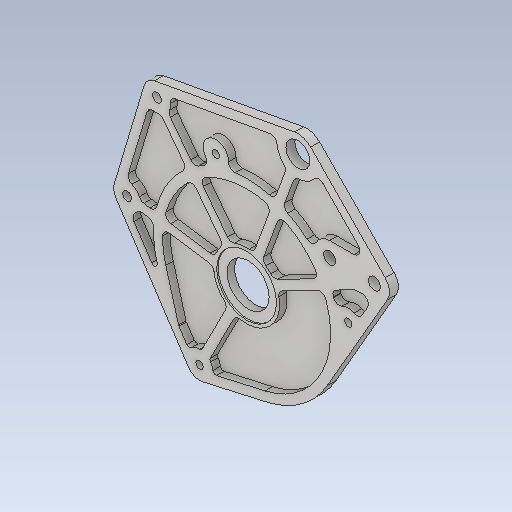
# Autodesk Inventor part: 前足内フレーム
Saved by Autodesk Inventor 2020 (Build 240168000, 168)
## iProperties
Created: 2019-09-17
Part Number: 前足内フレーム
Material: アルミニウム 2014-T4
Document SubType Name: Modeling
Designer: tanjihayato
Density: 2.8 g/cm^3
Appearance: サテン
Mass: 23.3541 g
Surface Area: 136.725 cm^2
Volume: 8.34073 cm^3
Author: tanjihayato
Autodesk Inventor part; units mm, degrees
note: some values were not read from the file. Chosen so that the rebuilt part matches the saved one: sketch regions of "押し出し9".
(part 1 of 2)
ref_plane "YZ Plane" through (0, 0, 0) normal (1, 0, 0) x (0, 1, 0)
ref_plane "XZ Plane" through (0, 0, 0) normal (0, 1, 0) x (-1, 0, 0)
ref_plane "XY Plane" through (0, 0, 0) normal (0, 0, 1) x (1, 0, 0)
sketch "スケッチ3" plane through (0, 0, 0) normal (0, 0, 1) x (1, 0, 0)
  circle A0 centre (110.4743, -16.4118) radius 30.1 construction
  circle A1 centre (150.4743, 0.5882) radius 1.5
  circle A2 centre (127.6431, 30.2622) radius 1.5
  circle A3 centre (80.4743, 23.124) radius 1.5
  circle A4 centre (70.4743, -10.4118) radius 1.5
  circle A5 centre (110.4743, -16.4118) radius 7.025
  arc A6 (79.801, 27.5733) -> (76.162, 24.4099) centre (80.4743, 23.124) ccw
  arc A7 (131.2097, 33.0062) -> (126.9698, 34.7115) centre (127.6431, 30.2622) ccw
  arc A8 (154.401, -1.6098) -> (154.0408, 3.3323) centre (150.4743, 0.5882) ccw
  arc A9 (66.162, -9.1259) -> (66.7172, -12.8885) centre (70.4743, -10.4118) ccw
  arc A10 (117.3199, -46.749) -> (137.6119, -31.6026) centre (110.4743, -16.4118) ccw
  line L0 (154.401, -1.6098) -> (137.6119, -31.6026)
  line L1 (66.162, -9.1259) -> (76.162, 24.4099)
  line L2 (79.801, 27.5733) -> (126.9698, 34.7115)
  line L3 (131.2097, 33.0062) -> (154.0408, 3.3323)
  line L4 (96.5433, 16.3458) -> (118.2214, -10.0492) construction
  line L5 (117.0311, -23.9953) -> (91.1935, -46.3348) construction
  circle A11 centre (100.1953, 16.6261) radius 3 construction
  circle A12 centre (144.4932, -10.0968) radius 3 construction
  circle A13 centre (100.1953, 16.6261) radius 4.5 construction
  circle A14 centre (144.4932, -10.0968) radius 4.5 construction
  arc A15 (90.988, -49.7066) -> (95.7356, -51.6195) centre (94.7451, -47.2298) ccw
  circle A16 centre (94.7451, -47.2298) radius 3 construction
  line L6 (95.7356, -51.6195) -> (117.3199, -46.749)
  line L7 (66.7172, -12.8885) -> (90.988, -49.7066)
  circle A17 centre (100.1953, 16.6261) radius 1.25
  circle A18 centre (144.4932, -10.0968) radius 1.25
  circle A19 centre (94.7451, -47.2298) radius 1.25
  circle A20 centre (110.4743, -16.4118) radius 30.1 construction
  circle A21 centre (150.4743, 0.5882) radius 1.5
  circle A22 centre (127.6431, 30.2622) radius 1.5
  circle A23 centre (80.4743, 23.124) radius 1.5
  circle A24 centre (70.4743, -10.4118) radius 1.5
  circle A25 centre (110.4743, -16.4118) radius 7.025
  arc A26 (79.801, 27.5733) -> (76.162, 24.4099) centre (80.4743, 23.124) ccw
  arc A27 (131.2097, 33.0062) -> (126.9698, 34.7115) centre (127.6431, 30.2622) ccw
  arc A28 (154.401, -1.6098) -> (154.0408, 3.3323) centre (150.4743, 0.5882) ccw
  arc A29 (66.162, -9.1259) -> (66.7172, -12.8885) centre (70.4743, -10.4118) ccw
  arc A30 (117.3199, -46.749) -> (137.6119, -31.6026) centre (110.4743, -16.4118) ccw
  line L8 (154.401, -1.6098) -> (137.6119, -31.6026)
  line L9 (66.162, -9.1259) -> (76.162, 24.4099)
  line L10 (79.801, 27.5733) -> (126.9698, 34.7115)
  line L11 (131.2097, 33.0062) -> (154.0408, 3.3323)
  line L12 (96.5433, 16.3458) -> (118.2214, -10.0492) construction
  line L13 (117.0311, -23.9953) -> (91.1935, -46.3348) construction
  circle A31 centre (100.1953, 16.6261) radius 3 construction
  circle A32 centre (144.4932, -10.0968) radius 3 construction
  circle A33 centre (100.1953, 16.6261) radius 4.5 construction
  circle A34 centre (144.4932, -10.0968) radius 4.5 construction
  arc A35 (90.988, -49.7066) -> (95.7356, -51.6195) centre (94.7451, -47.2298) ccw
  circle A36 centre (94.7451, -47.2298) radius 3 construction
  line L14 (95.7356, -51.6195) -> (117.3199, -46.749)
  line L15 (66.7172, -12.8885) -> (90.988, -49.7066)
  circle A37 centre (100.1953, 16.6261) radius 1.25
  circle A38 centre (144.4932, -10.0968) radius 1.25
  circle A39 centre (94.7451, -47.2298) radius 1.25
  circle A40 centre (153.2732, 5.5882) radius 1.5
  circle A41 centre (138.2732, 5.5882) radius 1.5
  arc A42 (157.1998, 3.3902) -> (156.3941, 8.8301) centre (153.2732, 5.5882) ccw
  line L16 (154.401, -1.6098) -> (157.1998, 3.3902)
  line L17 (130.7641, 33.504) -> (156.3941, 8.8301)
  circle A43 centre (138.2732, 5.5882) radius 3
  circle A44 centre (153.2732, 5.5882) radius 3
  point P0 (0, 0)
  point P1 (0, 0)
  point P2 (0, 0)
  dimension "d20" = 14.05
  dimension "d21" = 9
  dimension "d22" = 9
  dimension "d23" = 9
  dimension "d24" = 9
  dimension "d25" = 1
  dimension "d26" = 6
  dimension "d27" = 6
  dimension "d28" = 9
  dimension "d29" = 9
  dimension "d30" = 9
  dimension "d31" = 6
  dimension "d32" = 2.5
  dimension "d33" = 2.5
  dimension "d34" = 2.5
  dimension "d37" = 14.05
  dimension "d38" = 9
  dimension "d39" = 9
  dimension "d40" = 9
  dimension "d41" = 9
  dimension "d42" = 1
  dimension "d43" = 6
  dimension "d44" = 6
  dimension "d45" = 9
  dimension "d46" = 9
  dimension "d47" = 9
  dimension "d48" = 6
  dimension "d49" = 2.5
  dimension "d50" = 2.5
  dimension "d51" = 2.5
  dimension "d52" = 3
  dimension "d53" = 3
  dimension "d54" = 15
  dimension "d55" = 9
  dimension "d56" = 6
  dimension "d57" = 6
  dimension "d58" = 5
  constraints: 45 centre point, 39 tangent, 36 end point, 27 coincident, 27 point on circle, 1 collinear, 1 horizontal alignment
  measures "d20" diameter of A5
  measures "d21" diameter of A6
  measures "d22" diameter of A7
  measures "d23" diameter of A8
  measures "d24" diameter of A9
  measures "d25" radial gap between concentric circles of A10 A0
  measures "d26" diameter of A11
  measures "d27" diameter of A12
  measures "d28" diameter of A13
  measures "d29" diameter of A14
  measures "d30" diameter of A15
  measures "d31" diameter of A16
  measures "d32" diameter of A17
  measures "d33" diameter of A18
  measures "d34" diameter of A19
  measures "d37" diameter of A25
  measures "d38" diameter of A26
  measures "d39" diameter of A27
  measures "d40" diameter of A28
  measures "d41" diameter of A29
  measures "d42" radial gap between concentric circles of A30 A20
  measures "d43" diameter of A31
  measures "d44" diameter of A32
  measures "d45" diameter of A33
  measures "d46" diameter of A34
  measures "d47" diameter of A35
  measures "d48" diameter of A36
  measures "d49" diameter of A37
  measures "d50" diameter of A38
  measures "d51" diameter of A39
  measures "d52" diameter of A40
  measures "d53" diameter of A41
  measures "d54" distance of A41.centre A40.centre
  measures "d55" diameter of A42
  measures "d56" diameter of A43
  measures "d57" diameter of A44
  measures "d58" vertical distance of A21.centre A40.centre
extrude "押し出し3" add sketch "スケッチ3" along normal blind 3 contours A1 | L2 A7 L3 A44 A8 L0 A10 L6 A15 L7 A9 L1 A6 | L17 A42 L16 A8 A44 L3 A7 | A44 A8 L3 A40 | L3 A40 A8 A44 | A40 L3 | L3 A40 | A43
extrude "押し出し4" cut sketch "スケッチ3" along normal blind 10 contours A40 L3 | L3 A40
sketch "スケッチ4" plane through (0, 0, 3) normal (0, 0, 1) x (1, 0, 0)
  circle A0 centre (153.2732, 5.5882) radius 1.5 projected
  circle A1 centre (138.2732, 5.5882) radius 1.5 projected
  circle A2 centre (110.4743, -16.4118) radius 7.025 projected
  circle A3 centre (70.4743, -10.4118) radius 1.5 projected
  circle A4 centre (80.4743, 23.124) radius 1.5 projected
  circle A5 centre (127.6431, 30.2622) radius 1.5 projected
  circle A6 centre (94.7451, -47.2298) radius 1.25 projected
  circle A7 centre (144.4932, -10.0968) radius 1.25 projected
  circle A8 centre (100.1953, 16.6261) radius 1.25 projected
  arc A9 (79.801, 27.5733) -> (76.162, 24.4099) centre (80.4743, 23.124) ccw projected
  line L0 (76.162, 24.4099) -> (66.162, -9.1259) projected
  arc A10 (66.162, -9.1259) -> (66.7172, -12.8885) centre (70.4743, -10.4118) ccw projected
  line L1 (66.7172, -12.8885) -> (90.988, -49.7066) projected
  arc A11 (90.988, -49.7066) -> (95.7356, -51.6195) centre (94.7451, -47.2298) ccw projected
  line L2 (95.7356, -51.6195) -> (117.3199, -46.749) projected
  arc A12 (117.3199, -46.749) -> (137.6119, -31.6026) centre (110.4743, -16.4118) ccw projected
  line L3 (137.6119, -31.6026) -> (157.1998, 3.3902) projected
  arc A13 (157.1998, 3.3902) -> (156.3941, 8.8301) centre (153.2732, 5.5882) ccw projected
  line L4 (156.3941, 8.8301) -> (130.7641, 33.504) projected
  arc A14 (130.7641, 33.504) -> (126.9698, 34.7115) centre (127.6431, 30.2622) ccw projected
  line L5 (126.9698, 34.7115) -> (79.801, 27.5733) projected
  circle A15 centre (127.6431, 30.2622) radius 4.025
  arc A16 (131.983, 34.4054) -> (126.5593, 36.1635) centre (127.6431, 30.2622) ccw
  line L6 (79.6614, 27.5499) -> (126.5593, 36.1635)
  line L7 (131.983, 34.4054) -> (156.528, 8.6956)
  point P0 (0, 0)
  dimension "d61" = 8.05
  dimension "d62" = 12
  constraints: 4 end point, 4 point on circle, 4 tangent, 2 centre point, 2 coincident
  measures "d61" diameter of A15
  measures "d62" diameter of A16
extrude "押し出し5" add sketch "スケッチ4" against normal blind 3 contours A9 L6 A16 L7 A13 L4 A14 L5
extrude "押し出し6" cut sketch "スケッチ4" against normal blind 3 contours A15
sketch "スケッチ5" plane through (0, 0, 3) normal (0, 0, 1) x (1, 0, 0)
  circle A0 centre (127.6431, 30.2622) radius 4.025 projected
  circle A1 centre (153.2732, 5.5882) radius 1.5 projected
  circle A2 centre (138.2732, 5.5882) radius 1.5 projected
  circle A3 centre (110.4743, -16.4118) radius 7.025 projected
  circle A4 centre (70.4743, -10.4118) radius 1.5 projected
  circle A5 centre (80.4743, 23.124) radius 1.5 projected
  circle A6 centre (94.7451, -47.2298) radius 1.25 projected
  circle A7 centre (144.4932, -10.0968) radius 1.25 projected
  circle A8 centre (100.1953, 16.6261) radius 1.25 projected
  arc A9 (79.6614, 27.5499) -> (76.162, 24.4099) centre (80.4743, 23.124) ccw projected
  line L0 (76.162, 24.4099) -> (66.162, -9.1259) projected
  arc A10 (66.162, -9.1259) -> (66.7172, -12.8885) centre (70.4743, -10.4118) ccw projected
  line L1 (66.7172, -12.8885) -> (90.988, -49.7066) projected
  arc A11 (90.988, -49.7066) -> (95.7356, -51.6195) centre (94.7451, -47.2298) ccw projected
  line L2 (95.7356, -51.6195) -> (117.3199, -46.749) projected
  arc A12 (117.3199, -46.749) -> (137.6119, -31.6026) centre (110.4743, -16.4118) ccw projected
  line L3 (137.6119, -31.6026) -> (157.1998, 3.3902) projected
  arc A13 (157.1998, 3.3902) -> (156.528, 8.6956) centre (153.2732, 5.5882) ccw projected
  line L4 (156.528, 8.6956) -> (131.983, 34.4054) projected
  arc A14 (131.983, 34.4054) -> (126.5593, 36.1635) centre (127.6431, 30.2622) ccw projected
  line L5 (126.5593, 36.1635) -> (79.6614, 27.5499) projected
  circle A15 centre (153.2732, 5.5882) radius 2
  circle A16 centre (138.2732, 5.5882) radius 2
  arc A17 (157.6055, 3.092) -> (156.8408, 9.0914) centre (153.2732, 5.5882) ccw
  line L6 (131.9243, 34.466) -> (156.8408, 9.0914)
  line L7 (157.6055, 3.092) -> (137.4212, -31.9384)
  arc A18 (117.3199, -46.749) -> (137.6119, -31.6026) centre (110.4743, -16.4118) ccw projected
  arc A19 (131.983, 34.4054) -> (126.5593, 36.1635) centre (127.6431, 30.2622) ccw projected
  point P0 (0, 0)
  dimension "d67" = 4
  dimension "d68" = 4
  dimension "d69" = 3
  constraints: 4 end point, 4 point on circle, 4 tangent, 3 centre point, 2 coincident
  measures "d67" diameter of A15
  measures "d68" diameter of A16
  measures "d69" radial gap between concentric circles of A15 A17
extrude "押し出し7" add sketch "スケッチ5" against normal blind 3 contours L6 A17 L7 A12 L3 A13 L4
extrude "押し出し8" cut sketch "スケッチ5" against normal blind 3 contours A15 | A16
sketch "スケッチ6" plane through (0, 0, 3) normal (0, 0, 1) x (1, 0, 0)
  circle A0 centre (153.2732, 5.5882) radius 2 projected
  circle A1 centre (138.2732, 5.5882) radius 2 projected
  circle A2 centre (127.6431, 30.2622) radius 4.025 projected
  circle A3 centre (110.4743, -16.4118) radius 7.025 projected
  circle A4 centre (70.4743, -10.4118) radius 1.5 projected
  circle A5 centre (80.4743, 23.124) radius 1.5 projected
  circle A6 centre (94.7451, -47.2298) radius 1.25 projected
  circle A7 centre (144.4932, -10.0968) radius 1.25 projected
  circle A8 centre (100.1953, 16.6261) radius 1.25 projected
  arc A9 (79.6614, 27.5499) -> (76.162, 24.4099) centre (80.4743, 23.124) ccw projected
  line L0 (76.162, 24.4099) -> (66.162, -9.1259) projected
  arc A10 (66.162, -9.1259) -> (66.7172, -12.8885) centre (70.4743, -10.4118) ccw projected
  line L1 (66.7172, -12.8885) -> (90.988, -49.7066) projected
  arc A11 (90.988, -49.7066) -> (95.7356, -51.6195) centre (94.7451, -47.2298) ccw projected
  line L2 (95.7356, -51.6195) -> (117.3199, -46.749) projected
  arc A12 (117.3199, -46.749) -> (137.4212, -31.9384) centre (110.4743, -16.4118) ccw projected
  line L3 (137.4212, -31.9384) -> (157.6055, 3.092) projected
  arc A13 (157.6055, 3.092) -> (156.8408, 9.0914) centre (153.2732, 5.5882) ccw projected
  line L4 (156.8408, 9.0914) -> (131.9243, 34.466) projected
  arc A14 (131.9243, 34.466) -> (126.5593, 36.1635) centre (127.6431, 30.2622) ccw projected
  line L5 (126.5593, 36.1635) -> (79.6614, 27.5499) projected
  arc A15 (120.8535, 32.0653) -> (134.2343, 27.8317) centre (127.6431, 30.2622) ccw
  arc A16 (77.8245, 19.4869) -> (84.3762, 25.3657) centre (80.4743, 23.124) ccw
  arc A17 (71.557, -14.7796) -> (70.2492, -5.9174) centre (70.4743, -10.4118) ccw
  arc A18 (98.9543, -47.8178) -> (91.3042, -44.7354) centre (94.7451, -47.2298) ccw
  line L6 (153.2732, 5.5882) -> (138.2732, 5.5882) construction
  line L7 (151.1665, 10.5882) -> (138.2732, 10.5882)
  line L8 (138.2732, 0.5882) -> (152.7005, 0.5882)
  arc A19 (138.2732, 10.5882) -> (138.2732, 0.5882) centre (138.2732, 5.5882) ccw
  arc A20 (80.2034, 24.5993) -> (79.0369, 23.5526) centre (80.4743, 23.124) ccw
  line L9 (79.0369, 23.5526) -> (69.0369, -9.9832)
  arc A21 (69.0369, -9.9832) -> (69.222, -11.2374) centre (70.4743, -10.4118) ccw
  line L10 (69.222, -11.2374) -> (93.4928, -48.0554)
  arc A22 (93.4928, -48.0554) -> (95.0753, -48.6931) centre (94.7451, -47.2298) ccw
  line L11 (95.0753, -48.6931) -> (116.6595, -43.8226)
  arc A23 (116.6595, -43.8226) -> (134.8218, -30.4407) centre (110.4743, -16.4118) ccw
  line L12 (134.8218, -30.4407) -> (155.0061, 4.5897)
  arc A24 (155.0061, 4.5897) -> (154.7002, 6.9895) centre (153.2732, 5.5882) ccw
  line L13 (154.7002, 6.9895) -> (129.7837, 32.3641)
  arc A25 (129.7837, 32.3641) -> (127.1012, 33.2128) centre (127.6431, 30.2622) ccw
  line L14 (127.1012, 33.2128) -> (80.2034, 24.5993)
  circle A26 centre (100.1953, 16.6261) radius 4.25
  circle A27 centre (144.4932, -10.0968) radius 4.25
  circle A28 centre (110.4743, -16.4118) radius 11.025
  circle A29 centre (110.4743, -16.4118) radius 31.1
  circle A30 centre (110.4743, -16.4118) radius 28.1
  line L15 (127.6431, 30.2622) -> (110.4743, -16.4118) construction
  arc A31 (129.0509, 29.7443) -> (126.2354, 30.78) centre (127.6431, 30.2622) ccw
  arc A32 (109.0666, -15.894) -> (111.8821, -16.9296) centre (110.4743, -16.4118) ccw
  line L16 (80.4743, 23.124) -> (110.4743, -16.4118) construction
  arc A33 (81.6693, 24.0307) -> (79.2794, 22.2173) centre (80.4743, 23.124) ccw
  arc A34 (109.2794, -17.3185) -> (111.6693, -15.5051) centre (110.4743, -16.4118) ccw
  line L17 (94.7451, -47.2298) -> (110.4743, -16.4118) construction
  arc A35 (93.4091, -46.5479) -> (96.0812, -47.9118) centre (94.7451, -47.2298) ccw
  arc A36 (111.8104, -17.0937) -> (109.1383, -15.7299) centre (110.4743, -16.4118) ccw
  line L18 (153.2732, 5.5882) -> (110.4743, -16.4118) construction
  arc A37 (153.9589, 4.2541) -> (152.5874, 6.9223) centre (153.2732, 5.5882) ccw
  arc A38 (109.7886, -15.0777) -> (111.1601, -17.7459) centre (110.4743, -16.4118) ccw
  line L19 (70.4743, -10.4118) -> (110.4743, -16.4118) construction
  arc A39 (70.6968, -8.9284) -> (70.2518, -11.8952) centre (70.4743, -10.4118) ccw
  arc A40 (110.2518, -17.8952) -> (110.6968, -14.9284) centre (110.4743, -16.4118) ccw
  line L20 (111.1601, -17.7459) -> (111.5904, -17.5247)
  line L21 (117.2639, -14.6083) -> (153.9589, 4.2541)
  line L22 (152.5874, 6.9223) -> (115.8924, -11.9402)
  line L23 (113.2103, -13.3188) -> (109.7886, -15.0777)
  line L24 (111.8821, -16.9296) -> (113.2103, -13.3188)
  line L25 (114.2514, -10.4886) -> (129.0509, 29.7443)
  line L26 (126.2354, 30.78) -> (111.4359, -9.4529)
  line L27 (110.0127, -13.3219) -> (109.0666, -15.894)
  line L28 (111.6693, -15.5051) -> (110.0127, -13.3219)
  line L29 (107.5207, -10.0379) -> (81.6693, 24.0307)
  line L30 (79.2794, 22.2173) -> (105.1309, -11.8513)
  line L31 (107.0508, -14.3815) -> (109.2794, -17.3185)
  line L32 (110.6968, -14.9284) -> (107.0508, -14.3815)
  line L33 (103.9098, -13.9103) -> (70.6968, -8.9284)
  line L34 (70.2518, -11.8952) -> (103.4648, -16.8771)
  line L35 (108.1909, -17.5861) -> (110.2518, -17.8952)
  line L36 (109.1383, -15.7299) -> (108.1909, -17.5861)
  line L37 (106.0184, -21.8427) -> (93.4091, -46.5479)
  line L38 (96.0812, -47.9118) -> (108.6904, -23.2065)
  line L39 (111.5904, -17.5247) -> (111.8104, -17.0937)
  circle A41 centre (110.4743, -16.4118) radius 10
  point P0 (0, 0)
  point P1 (145.7732, 5.5882)
  point P2 (119.0587, 6.9252)
  point P3 (95.4743, 3.3561)
  point P4 (102.6097, -31.8208)
  point P5 (131.8738, -5.4118)
  point P6 (90.4743, -13.4118)
  dimension "d74" = 10
  dimension "d75" = 3
  dimension "d76" = 3
  dimension "d77" = 3
  dimension "d78" = 3
  dimension "d79" = 3
  dimension "d80" = 3
  dimension "d81" = 3
  dimension "d82" = 4
  dimension "d83" = 3
  dimension "d84" = 3
  dimension "d85" = 3
  dimension "d86" = 3
  dimension "d87" = 3
  dimension "d100" = 20
  constraints: 80 end point, 42 point on circle, 42 tangent, 27 centre point, 21 parallel, 10 point on line, 7 coincident, 6 midpoint, 5 concentric, 2 horizontal, 22 other
  measures "d74" diameter of A19
  measures "d75" distance between parallel lines of L5 L14
  measures "d76" radial gap between concentric circles of A8 A26
  measures "d77" radial gap between concentric circles of A7 A27
  measures "d78" radial gap between concentric circles of A16 A5
  measures "d79" radial gap between concentric circles of A17 A4
  measures "d80" radial gap between concentric circles of A18 A6
  measures "d81" radial gap between concentric circles of A15 A2
  measures "d83" diameter of A32
  measures "d84" diameter of A34
  measures "d85" diameter of A36
  measures "d86" diameter of A38
  measures "d87" diameter of A40
  measures "d100" diameter of A41
extrude "押し出し9" cut sketch "スケッチ6" against normal blind 10 contours L7 A19 A29 L25 A15 L13 | L12 A27 A29 L21 L8 | L22 A29 A19 L8 | L8 L21 A29 L22 | L12 A27 A29 | L22 A30 L25 A29 A19 | A29 L21 A30 L22 | L25 A29 L26 A15 | A29 A27 L12 A30 L21 | L12 A29 A27 | A29 A27 | L22 A28 L25 A30 | A30 L21 A28 L22 | L25 A30 L26 A29 | L26 A29 A26 L29 A16 L14 A15 | A30 A23 L38 A28 L21 | L25 A28 L26 A30 | L26 A30 L29 A29 A26 | L26 A28 L29 A30 | L11 A29 A18 L38 A30 | L29 A28 L30 A30 | A30 L30 A29 L29 | L29 A29 L30 A16 | L38 A30 L37 A28 | L11 A18 A29 | L38 A18 L37 A30 | L30 A28 L33 A30 | A30 L33 A29 L30 | L30 A29 L33 A17 L9 A16 | L37 A30 L34 A28 | L37 A18 A29 L34 A30 | L33 A28 L34 A30 | A30 L34 A29 L33 | A29 L34 A17 L33 | A29 A18 L10 A17 L34
extrude "押し出し10" add sketch "スケッチ6" against normal blind 3 contours L22 A37 L21 A0 | A0 L21 L8 L22 | L8 L21 A29 L22 | A27 L12 | L12 A27 A29 | L22 A30 L25 A29 A19 | A29 L21 A30 L22 | A29 A19 | L25 A29 L26 A15 | A15 L26 A2 L25 | A29 A27 L12 A30 L21 | A29 A27 | A30 L21 A28 L22 | L25 A30 L26 A29 | A2 L26 A31 L25 | A29 A12 L11 A23 L12 | L25 A28 L26 A30 | A28 L21 A41 L22 | L26 A30 L29 A29 A26 | L25 A41 L26 A28 | A41 L21 A3 L22 | A26 A29 | L11 A29 A18 L38 A30 | L29 A28 L30 A30 | A30 L30 A29 L29 | L25 A3 L26 A41 | L29 A29 L30 A16 | A16 L30 A5 L29 | L38 A30 L37 A28 | A28 L37 A41 L38 | L38 A18 L37 A30 | A30 L33 A29 L30 | L29 A41 L30 A28 | A41 L37 A3 L38 | A29 L38 A18 | L37 A18 A29 L34 A30 | L38 A29 L37 A18 | L33 A28 L34 A30 | A30 L34 A29 L33 | L29 A3 L30 A41 | A28 L33 A41 L34 | A22 A35 L37 A29 L38 | L37 A29 A18 | A29 L34 A17 L33 | A41 L33 A3 L34 | A17 L34 A4 L33 picked at (152.6478, 5.3573) picked at (145.8885, -10.8818) picked at (101.4617, 13.0958)
extrude "押し出し11" cut sketch "スケッチ6" against normal blind 3 contours A0 L21 A37 L22 | L22 A37 L21 A0 | L13 A25 L14 A2 | A2 L25 A31 L26 L14 A25 L13 | A2 L26 A31 L25
sketch "スケッチ7" plane through (0, 0, 3) normal (0, 0, 1) x (1, 0, 0)
  circle A0 centre (153.2732, 5.5882) radius 2 projected
  circle A1 centre (127.6431, 30.2622) radius 4.025 projected
  line L0 (144.1052, -14.3291) -> (141.4751, -18.8937) projected
  arc A2 (141.4751, -18.8937) -> (141.3863, -12.9968) centre (110.4743, -16.4118) ccw projected
  arc A3 (141.3863, -12.9968) -> (144.1052, -14.3291) centre (144.4932, -10.0968) ccw projected
  arc A4 (136.2251, 1.0269) -> (138.2732, 0.5882) centre (138.2732, 5.5882) ccw projected
  line L1 (138.2732, 0.5882) -> (140.2651, 0.5882) projected
  line L2 (140.2651, 0.5882) -> (137.4161, -0.8763) projected
  arc A5 (137.4161, -0.8763) -> (136.2251, 1.0269) centre (110.4743, -16.4118) ccw projected
  arc A6 (94.3399, -42.9992) -> (91.3042, -44.7354) centre (94.7451, -47.2298) ccw projected
  line L3 (91.3042, -44.7354) -> (71.557, -14.7796) projected
  arc A7 (71.557, -14.7796) -> (74.4475, -12.5246) centre (70.4743, -10.4118) ccw projected
  line L4 (74.4475, -12.5246) -> (79.5317, -13.2872) projected
  arc A8 (79.5317, -13.2872) -> (94.3399, -42.9992) centre (110.4743, -16.4118) ccw projected
  arc A9 (147.9602, -7.6387) -> (140.5525, -8.5052) centre (144.4932, -10.0968) ccw projected
  arc A10 (140.5525, -8.5052) -> (138.7876, -3.5444) centre (110.4743, -16.4118) ccw projected
  line L5 (138.7876, -3.5444) -> (146.8272, 0.5882) projected
  line L6 (146.8272, 0.5882) -> (152.7005, 0.5882) projected
  line L7 (152.7005, 0.5882) -> (147.9602, -7.6387) projected
  arc A11 (99.0543, -42.0865) -> (136.116, -4.9177) centre (110.4743, -16.4118) ccw projected
  line L8 (99.0543, -42.0865) -> (106.845, -26.8223) projected
  arc A12 (106.845, -26.8223) -> (120.8743, -12.7524) centre (110.4743, -16.4118) ccw projected
  line L9 (120.8743, -12.7524) -> (136.116, -4.9177) projected
  arc A13 (98.4089, -45.076) -> (103.6597, -46.756) centre (110.4743, -16.4118) ccw projected
  line L10 (103.6597, -46.756) -> (98.9543, -47.8178) projected
  arc A14 (98.9543, -47.8178) -> (98.4089, -45.076) centre (94.7451, -47.2298) ccw projected
  arc A15 (133.3633, 4.643) -> (122.6063, 12.2243) centre (110.4743, -16.4118) ccw projected
  line L11 (122.6063, 12.2243) -> (126.6816, 23.3033) projected
  arc A16 (126.6816, 23.3033) -> (134.2343, 27.8317) centre (127.6431, 30.2622) ccw projected
  line L12 (134.2343, 27.8317) -> (151.1665, 10.5882) projected
  line L13 (151.1665, 10.5882) -> (138.2732, 10.5882) projected
  arc A17 (138.2732, 10.5882) -> (133.3633, 4.643) centre (138.2732, 5.5882) ccw projected
  arc A18 (74.8925, -9.5578) -> (70.2492, -5.9174) centre (70.4743, -10.4118) ccw projected
  line L14 (70.2492, -5.9174) -> (77.8245, 19.4869) projected
  arc A19 (77.8245, 19.4869) -> (81.844, 18.8375) centre (80.4743, 23.124) ccw projected
  line L15 (81.844, 18.8375) -> (90.5019, 7.4275) projected
  arc A20 (90.5019, 7.4275) -> (79.9767, -10.3204) centre (110.4743, -16.4118) ccw projected
  line L16 (79.9767, -10.3204) -> (74.8925, -9.5578) projected
  line L17 (104.1729, -25.4585) -> (96.3822, -40.7227) projected
  arc A21 (82.5023, -13.7328) -> (96.3822, -40.7227) centre (110.4743, -16.4118) ccw projected
  line L18 (82.5023, -13.7328) -> (99.4502, -16.275) projected
  arc A22 (99.4502, -16.275) -> (104.1729, -25.4585) centre (110.4743, -16.4118) ccw projected
  circle A23 centre (110.4743, -16.4118) radius 7.025 projected
  circle A24 centre (144.4932, -10.0968) radius 1.25 projected
  circle A25 centre (100.1953, 16.6261) radius 1.25 projected
  arc A26 (102.677, -8.6175) -> (99.8952, -13.3081) centre (110.4743, -16.4118) ccw projected
  line L19 (99.8952, -13.3081) -> (82.9474, -10.766) projected
  arc A27 (92.3177, 5.0346) -> (82.9474, -10.766) centre (110.4743, -16.4118) ccw projected
  line L20 (92.3177, 5.0346) -> (102.677, -8.6175) projected
  line L21 (115.6529, -6.6787) -> (121.5692, 9.4051) projected
  arc A28 (134.7445, -2.2496) -> (121.5692, 9.4051) centre (110.4743, -16.4118) ccw projected
  line L22 (134.7445, -2.2496) -> (119.5028, -10.0843) projected
  arc A29 (119.5028, -10.0843) -> (115.6529, -6.6787) centre (110.4743, -16.4118) ccw projected
  arc A30 (112.8373, -5.643) -> (105.0668, -6.804) centre (110.4743, -16.4118) ccw projected
  line L23 (105.0668, -6.804) -> (94.7076, 6.848) projected
  arc A31 (118.7537, 10.4408) -> (94.7076, 6.848) centre (110.4743, -16.4118) ccw projected
  line L24 (118.7537, 10.4408) -> (112.8373, -5.643) projected
  circle A32 centre (94.7451, -47.2298) radius 1.25 projected
  line L25 (123.8661, 24.339) -> (119.7907, 13.26) projected
  arc A33 (119.7907, 13.26) -> (103.4411, 13.8825) centre (110.4743, -16.4118) ccw projected
  arc A34 (103.4411, 13.8825) -> (99.079, 12.5253) centre (100.1953, 16.6261) ccw projected
  arc A35 (99.079, 12.5253) -> (92.8918, 9.241) centre (110.4743, -16.4118) ccw projected
  line L26 (92.8918, 9.241) -> (84.2339, 20.6509) projected
  arc A36 (84.2339, 20.6509) -> (84.3762, 25.3657) centre (80.4743, 23.124) ccw projected
  line L27 (84.3762, 25.3657) -> (120.8535, 32.0653) projected
  arc A37 (120.8535, 32.0653) -> (123.8661, 24.339) centre (127.6431, 30.2622) ccw projected
  arc A38 (117.3199, -46.749) -> (137.4212, -31.9384) centre (110.4743, -16.4118) ccw projected
  line L28 (137.4212, -31.9384) -> (157.6055, 3.092) projected
  arc A39 (157.6055, 3.092) -> (156.8408, 9.0914) centre (153.2732, 5.5882) ccw projected
  line L29 (156.8408, 9.0914) -> (131.9243, 34.466) projected
  arc A40 (131.9243, 34.466) -> (126.5593, 36.1635) centre (127.6431, 30.2622) ccw projected
  line L30 (126.5593, 36.1635) -> (79.6614, 27.5499) projected
  arc A41 (79.6614, 27.5499) -> (76.162, 24.4099) centre (80.4743, 23.124) ccw projected
  line L31 (76.162, 24.4099) -> (66.162, -9.1259) projected
  arc A42 (66.162, -9.1259) -> (66.7172, -12.8885) centre (70.4743, -10.4118) ccw projected
  line L32 (66.7172, -12.8885) -> (90.988, -49.7066) projected
  arc A43 (90.988, -49.7066) -> (95.7356, -51.6195) centre (94.7451, -47.2298) ccw projected
  line L33 (95.7356, -51.6195) -> (117.3199, -46.749) projected
  circle A44 centre (80.4743, 23.124) radius 1.5 projected
  circle A45 centre (138.2732, 5.5882) radius 2 projected
  circle A46 centre (70.4743, -10.4118) radius 1.5 projected
  arc A47 (78.7483, -25.6886) -> (80.5456, -24.8663) centre (79.5832, -25.1382) ccw
  line L34 (91.3042, -44.7354) -> (71.557, -14.7796) projected
  point P0 (0, 0)
  dimension "d94" = 2
  constraints: 3 point on circle, 2 tangent, 1 centre point, 1 point on line
  measures "d94" diameter of A47
extrude "押し出し12" add sketch "スケッチ7" against normal blind 3 contours L0 A2 A3 | A4 L1 L2 A5 | A6 L3 A47 A8 | A13 L10 A14
fillet "フィレット1" radius 2 47 edges at (152.7005, 0.5882, 1.5) (147.9602, -7.6387, 1.5) (146.8272, 0.5882, 1.5) (133.3633, 4.643, 1.5) (151.1665, 10.5882, 1.5) (134.2343, 27.8317, 1.5) (126.6816, 23.3033, 1.5) (120.8535, 32.0653, 1.5) (123.8661, 24.339, 1.5) (84.3762, 25.3657, 1.5) (84.2339, 20.6509, 1.5) (77.8245, 19.4869, 1.5) (81.844, 18.8375, 1.5) (70.2492, -5.9174, 1.5) (74.8925, -9.5578, 1.5) (71.557, -14.7796, 1.5) (74.4475, -12.5246, 1.5) (140.5525, -8.5052, 1.5) (138.7876, -3.5444, 1.5) (122.6063, 12.2243, 1.5) (119.7907, 13.26, 1.5) (92.8918, 9.241, 1.5) (90.5019, 7.4275, 1.5) (79.9767, -10.3204, 1.5) (79.5317, -13.2872, 1.5) (136.116, -4.9177, 1.5) (120.8743, -12.7524, 1.5) (119.5028, -10.0843, 1.5) (134.7445, -2.2496, 1.5) (121.5692, 9.4051, 1.5) (115.6529, -6.6787, 1.5) (112.8373, -5.643, 1.5) (118.7537, 10.4408, 1.5) (94.7076, 6.848, 1.5) (105.0668, -6.804, 1.5) (102.677, -8.6175, 1.5) (92.3177, 5.0346, 1.5) (82.9474, -10.766, 1.5) (99.8952, -13.3081, 1.5) (99.4502, -16.275, 1.5) (82.5023, -13.7328, 1.5) (96.3822, -40.7227, 1.5) (104.1729, -25.4585, 1.5) (106.845, -26.8223, 1.5) (99.0543, -42.0865, 1.5) (99.079, 12.5253, 1.5) (103.4411, 13.8825, 1.5)
sketch "スケッチ8" plane through (0, 0, 0) normal (0, 0, -1) x (-1, 0, 0)
  line L0 (-149.151, -5.572) -> (-150.9727, -2.4103) projected
  arc A0 (-149.2398, 0.5882) -> (-150.9727, -2.4103) centre (-149.2398, -1.4118) ccw projected
  line L1 (-149.2398, 0.5882) -> (-147.3112, 0.5882) projected
  arc A1 (-146.3968, 0.367) -> (-147.3112, 0.5882) centre (-147.3112, -1.4118) ccw projected
  line L2 (-146.3968, 0.367) -> (-140.4335, -2.6984) projected
  arc A2 (-139.4824, -5.1983) -> (-140.4335, -2.6984) centre (-141.3478, -4.4771) ccw projected
  arc A3 (-139.4824, -5.1983) -> (-139.547, -5.3668) centre (-110.4743, -16.4118) ccw projected
  arc A4 (-142.4011, -6.3974) -> (-139.547, -5.3668) centre (-141.4166, -4.6565) ccw projected
  arc A5 (-142.4011, -6.3974) -> (-146.4821, -6.341) centre (-144.4932, -10.0968) ccw projected
  arc A6 (-149.151, -5.572) -> (-146.4821, -6.341) centre (-147.4181, -4.5735) ccw projected
  arc A7 (-133.802, 7.8261) -> (-138.2732, 10.5882) centre (-138.2732, 5.5882) ccw projected
  line L3 (-138.2732, 10.5882) -> (-146.3996, 10.5882) projected
  arc A8 (-147.8266, 13.9895) -> (-146.3996, 10.5882) centre (-146.3996, 12.5882) ccw projected
  line L4 (-147.8266, 13.9895) -> (-136.068, 25.9642) projected
  arc A9 (-133.0902, 25.8259) -> (-136.068, 25.9642) centre (-134.641, 24.563) ccw projected
  arc A10 (-133.0902, 25.8259) -> (-127.9646, 23.2445) centre (-127.6431, 30.2622) ccw projected
  arc A11 (-126.1791, 21.9371) -> (-127.9646, 23.2445) centre (-128.0561, 21.2466) ccw projected
  line L5 (-126.1791, 21.9371) -> (-123.2452, 13.9611) projected
  arc A12 (-124.2371, 11.4772) -> (-123.2452, 13.9611) centre (-125.1222, 13.2707) ccw projected
  arc A13 (-124.2371, 11.4772) -> (-130.712, 7.2027) centre (-110.4743, -16.4118) ccw projected
  arc A14 (-133.802, 7.8261) -> (-130.712, 7.2027) centre (-132.0135, 8.7213) ccw projected
  arc A15 (-136.9629, -7.0327) -> (-101.1717, -42.9273) centre (-110.4743, -16.4118) ccw projected
  arc A16 (-134.1632, -5.9215) -> (-136.9629, -7.0327) centre (-135.0776, -7.7003) ccw projected
  line L6 (-134.1632, -5.9215) -> (-122.3182, -12.0102) projected
  arc A17 (-121.2735, -14.1917) -> (-122.3182, -12.0102) centre (-123.2325, -13.789) ccw projected
  arc A18 (-121.2735, -14.1917) -> (-108.2854, -27.2173) centre (-110.4743, -16.4118) ccw projected
  arc A19 (-106.107, -28.2683) -> (-108.2854, -27.2173) centre (-107.8884, -29.1775) ccw projected
  line L7 (-106.107, -28.2683) -> (-100.0524, -40.1309) projected
  arc A20 (-101.1717, -42.9273) -> (-100.0524, -40.1309) centre (-101.8338, -41.0401) ccw projected
  arc A21 (-122.8508, 25.1256) -> (-120.6357, 29.7665) centre (-127.6431, 30.2622) ccw projected
  arc A22 (-118.2794, 31.5925) -> (-120.6357, 29.7665) centre (-118.6406, 29.6254) ccw projected
  line L8 (-118.2794, 31.5925) -> (-86.5775, 25.77) projected
  arc A23 (-84.9497, 23.594) -> (-86.5775, 25.77) centre (-86.9388, 23.8029) ccw projected
  arc A24 (-84.9497, 23.594) -> (-84.6967, 21.568) centre (-80.4743, 23.124) ccw projected
  arc A25 (-84.9801, 19.6674) -> (-84.6967, 21.568) centre (-86.5734, 20.8764) ccw projected
  line L9 (-84.9801, 19.6674) -> (-91.7731, 10.7152) projected
  arc A26 (-94.4001, 10.212) -> (-91.7731, 10.7152) centre (-93.3664, 11.9242) ccw projected
  arc A27 (-94.4001, 10.212) -> (-96.0809, 11.157) centre (-110.4743, -16.4118) ccw projected
  arc A28 (-96.7681, 14.1127) -> (-96.0809, 11.157) centre (-95.1553, 12.9299) ccw projected
  arc A29 (-96.7681, 14.1127) -> (-104.4434, 16.5007) centre (-100.1953, 16.6261) ccw projected
  arc A30 (-106.6862, 14.4566) -> (-104.4434, 16.5007) centre (-106.4426, 16.4417) ccw projected
  arc A31 (-106.6862, 14.4566) -> (-118.0645, 13.7478) centre (-110.4743, -16.4118) ccw projected
  arc A32 (-120.4296, 14.9968) -> (-118.0645, 13.7478) centre (-118.5526, 15.6873) ccw projected
  line L10 (-120.4296, 14.9968) -> (-123.3635, 22.9728) projected
  arc A33 (-122.8508, 25.1256) -> (-123.3635, 22.9728) centre (-121.4865, 23.6632) ccw projected
  arc A34 (-80.5456, -24.8663) -> (-79.403, -15.0764) centre (-110.4743, -16.4118) ccw projected
  arc A35 (-77.7015, -13.0127) -> (-79.403, -15.0764) centre (-77.4049, -14.9905) ccw projected
  line L11 (-77.7015, -13.0127) -> (-75.6684, -12.7077) projected
  arc A36 (-73.8649, -13.3706) -> (-75.6684, -12.7077) centre (-75.3718, -14.6856) ccw projected
  arc A37 (-73.8649, -13.3706) -> (-73.2327, -13.9673) centre (-70.4743, -10.4118) ccw projected
  arc A38 (-72.7888, -16.6482) -> (-73.2327, -13.9673) centre (-74.4587, -15.5475) ccw projected
  line L12 (-72.7888, -16.6482) -> (-78.7483, -25.6886) projected
  arc A39 (-80.5456, -24.8663) -> (-78.7483, -25.6886) centre (-79.5832, -25.1382) ccw projected
  circle A40 centre (-110.4743, -16.4118) radius 7.025 projected
  line L13 (-101.6956, -7.3242) -> (-93.645, 3.2855) projected
  arc A41 (-90.64, 3.4932) -> (-93.645, 3.2855) centre (-92.0517, 2.0765) ccw projected
  arc A42 (-83.4952, -8.5546) -> (-90.64, 3.4932) centre (-110.4743, -16.4118) ccw projected
  arc A43 (-85.1187, -11.0917) -> (-83.4952, -8.5546) centre (-85.4154, -9.1138) ccw projected
  line L14 (-85.1187, -11.0917) -> (-98.2897, -13.0673) projected
  arc A44 (-100.4118, -11.9067) -> (-98.2897, -13.0673) centre (-98.5864, -11.0895) ccw projected
  arc A45 (-100.4118, -11.9067) -> (-101.695, -9.7429) centre (-110.4743, -16.4118) ccw projected
  arc A46 (-101.6956, -7.3242) -> (-101.695, -9.7429) centre (-100.1024, -8.5331) ccw projected
  circle A47 centre (-144.4932, -10.0968) radius 1.25 projected
  circle A48 centre (-100.1953, 16.6261) radius 1.25 projected
  arc A49 (-103.0079, -24.5237) -> (-99.5329, -17.7663) centre (-110.4743, -16.4118) ccw projected
  arc A50 (-97.8447, -16.0341) -> (-99.5329, -17.7663) centre (-97.548, -18.012) ccw projected
  line L15 (-97.8447, -16.0341) -> (-84.6737, -14.0585) projected
  arc A51 (-82.3772, -16.0076) -> (-84.6737, -14.0585) centre (-84.377, -16.0364) ccw projected
  arc A52 (-94.4591, -39.5012) -> (-82.3772, -16.0076) centre (-110.4743, -16.4118) ccw projected
  arc A53 (-97.3804, -38.7671) -> (-94.4591, -39.5012) centre (-95.599, -37.8579) ccw projected
  line L16 (-97.3804, -38.7671) -> (-103.4349, -26.9045) projected
  arc A54 (-103.0079, -24.5237) -> (-103.4349, -26.9045) centre (-101.6535, -25.9953) ccw projected
  line L17 (-113.3978, -4.1194) -> (-117.9957, 8.3801) projected
  arc A55 (-116.5511, 11.0233) -> (-117.9957, 8.3801) centre (-116.1186, 9.0706) ccw projected
  arc A56 (-96.6437, 8.0488) -> (-116.5511, 11.0233) centre (-110.4743, -16.4118) ccw projected
  arc A57 (-96.0348, 5.0989) -> (-96.6437, 8.0488) centre (-97.6281, 6.3079) ccw projected
  line L18 (-96.0348, 5.0989) -> (-104.0855, -5.5107) projected
  arc A58 (-106.4151, -6.1613) -> (-104.0855, -5.5107) centre (-105.6787, -4.3018) ccw projected
  arc A59 (-106.4151, -6.1613) -> (-111.3601, -5.4224) centre (-110.4743, -16.4118) ccw projected
  arc A60 (-113.3978, -4.1194) -> (-111.3601, -5.4224) centre (-111.5208, -3.4289) ccw projected
  arc A61 (-116.9209, -7.468) -> (-118.5647, -8.922) centre (-110.4743, -16.4118) ccw projected
  arc A62 (-120.9467, -9.3421) -> (-118.5647, -8.922) centre (-120.0323, -7.5633) ccw projected
  line L19 (-120.9467, -9.3421) -> (-132.7917, -3.2534) projected
  arc A63 (-133.5175, -0.33) -> (-132.7917, -3.2534) centre (-131.8774, -1.4746) ccw projected
  arc A64 (-123.6242, 8.4215) -> (-133.5175, -0.33) centre (-110.4743, -16.4118) ccw projected
  arc A65 (-120.8112, 7.3444) -> (-123.6242, 8.4215) centre (-122.6883, 6.654) ccw projected
  line L20 (-120.8112, 7.3444) -> (-116.2133, -5.1551) projected
  arc A66 (-116.9209, -7.468) -> (-116.2133, -5.1551) centre (-118.0904, -5.8455) ccw projected
  circle A67 centre (-94.7451, -47.2298) radius 1.25 projected
  circle A68 centre (-153.2732, 5.5882) radius 2 projected
  line L21 (-76.1135, -9.7409) -> (-78.1466, -10.0459) projected
  arc A69 (-80.3787, -8.5721) -> (-78.1466, -10.0459) centre (-78.4432, -8.068) ccw projected
  arc A70 (-80.3787, -8.5721) -> (-89.1607, 6.2363) centre (-110.4743, -16.4118) ccw projected
  arc A71 (-89.3833, 8.9018) -> (-89.1607, 6.2363) centre (-87.79, 7.6928) ccw projected
  line L22 (-89.3833, 8.9018) -> (-82.5903, 17.854) projected
  arc A72 (-80.8362, 18.6385) -> (-82.5903, 17.854) centre (-80.997, 16.645) ccw projected
  arc A73 (-80.8362, 18.6385) -> (-79.524, 18.7255) centre (-80.4743, 23.124) ccw projected
  arc A74 (-77.185, 17.3421) -> (-79.524, 18.7255) centre (-79.1016, 16.7706) ccw projected
  line L23 (-77.185, 17.3421) -> (-70.8888, -3.7727) projected
  arc A75 (-72.0881, -6.2111) -> (-70.8888, -3.7727) centre (-72.8054, -4.3442) ccw projected
  arc A76 (-72.0881, -6.2111) -> (-74.5837, -8.578) centre (-70.4743, -10.4118) ccw projected
  arc A77 (-76.1135, -9.7409) -> (-74.5837, -8.578) centre (-76.4101, -7.763) ccw projected
  circle A78 centre (-127.6431, 30.2622) radius 4.025 projected
  circle A79 centre (-70.4743, -10.4118) radius 1.5 projected
  arc A80 (-137.4212, -31.9384) -> (-117.3199, -46.749) centre (-110.4743, -16.4118) ccw projected
  line L24 (-95.7356, -51.6195) -> (-117.3199, -46.749) projected
  arc A81 (-95.7356, -51.6195) -> (-90.988, -49.7066) centre (-94.7451, -47.2298) ccw projected
  line L25 (-66.7172, -12.8885) -> (-90.988, -49.7066) projected
  arc A82 (-66.7172, -12.8885) -> (-66.162, -9.1259) centre (-70.4743, -10.4118) ccw projected
  line L26 (-76.162, 24.4099) -> (-66.162, -9.1259) projected
  arc A83 (-76.162, 24.4099) -> (-79.6614, 27.5499) centre (-80.4743, 23.124) ccw projected
  line L27 (-79.6614, 27.5499) -> (-126.5593, 36.1635) projected
  arc A84 (-126.5593, 36.1635) -> (-131.9243, 34.466) centre (-127.6431, 30.2622) ccw projected
  line L28 (-131.9243, 34.466) -> (-156.8408, 9.0914) projected
  arc A85 (-156.8408, 9.0914) -> (-157.6055, 3.092) centre (-153.2732, 5.5882) ccw projected
  line L29 (-157.6055, 3.092) -> (-137.4212, -31.9384) projected
  circle A86 centre (-80.4743, 23.124) radius 1.5 projected
  circle A87 centre (-138.2732, 5.5882) radius 2 projected
  point P0 (0, 0)
extrude "押し出し13" add sketch "スケッチ8" against normal blind 0.5 contours L0 A0 L1 A1 L2 A2 A3 A4 A5 A6 | A7 L3 A8 L4 A9 A10 A11 L5 A12 A13 A14 | A16 L6 A17 A18 A19 L7 A20 A15 | A21 A22 L8 A23 A24 A25 L9 A26 A27 A28 A29 A30 A31 A32 L10 A33 | A34 A35 L11 A36 A37 A38 L12 A39 | L13 A41 A42 A43 L14 A44 A45 A46 | A49 A50 L15 A51 A52 A53 L16 A54 | L17 A55 A56 A57 L18 A58 A59 A60 | A61 A62 L19 A63 A64 A65 L20 A66 | L21 A69 A70 A71 L22 A72 A73 A74 L23 A75 A76 A77
extrude "押し出し14" cut sketch "スケッチ6" against normal blind 0.5 contours A41 L21 A3 L22 | L22 A3 L25 A41 | A41 L38 A3 L21 | L25 A3 L26 A41 | L26 A3 L29 A41 | A41 L37 A3 L38 | L29 A3 L30 A41 | A41 L34 A3 L37 | L30 A3 L33 A41 | A41 L33 A3 L34
sketch "スケッチ9" plane through (0, 0, 3) normal (0, 0, 1) x (1, 0, 0)
  circle A0 centre (110.4743, -16.4118) radius 10 projected
  circle A1 centre (153.2732, 5.5882) radius 2 projected
  circle A2 centre (127.6431, 30.2622) radius 4.025 projected
  arc A3 (78.7483, -25.6886) -> (80.5456, -24.8663) centre (79.5832, -25.1382) ccw projected
  line L0 (78.7483, -25.6886) -> (72.7888, -16.6482) projected
  arc A4 (73.2327, -13.9673) -> (72.7888, -16.6482) centre (74.4587, -15.5475) ccw projected
  arc A5 (73.2327, -13.9673) -> (73.8649, -13.3706) centre (70.4743, -10.4118) ccw projected
  arc A6 (75.6684, -12.7077) -> (73.8649, -13.3706) centre (75.3718, -14.6856) ccw projected
  line L1 (75.6684, -12.7077) -> (77.7015, -13.0127) projected
  arc A7 (79.403, -15.0764) -> (77.7015, -13.0127) centre (77.4049, -14.9905) ccw projected
  arc A8 (79.403, -15.0764) -> (80.5456, -24.8663) centre (110.4743, -16.4118) ccw projected
  line L2 (140.4335, -2.6984) -> (146.3968, 0.367) projected
  arc A9 (147.3112, 0.5882) -> (146.3968, 0.367) centre (147.3112, -1.4118) ccw projected
  line L3 (147.3112, 0.5882) -> (149.2398, 0.5882) projected
  arc A10 (150.9727, -2.4103) -> (149.2398, 0.5882) centre (149.2398, -1.4118) ccw projected
  line L4 (150.9727, -2.4103) -> (149.151, -5.572) projected
  arc A11 (146.4821, -6.341) -> (149.151, -5.572) centre (147.4181, -4.5735) ccw projected
  arc A12 (146.4821, -6.341) -> (142.4011, -6.3974) centre (144.4932, -10.0968) ccw projected
  arc A13 (139.547, -5.3668) -> (142.4011, -6.3974) centre (141.4166, -4.6565) ccw projected
  arc A14 (139.547, -5.3668) -> (139.4824, -5.1983) centre (110.4743, -16.4118) ccw projected
  arc A15 (140.4335, -2.6984) -> (139.4824, -5.1983) centre (141.3478, -4.4771) ccw projected
  arc A16 (101.1717, -42.9273) -> (136.9629, -7.0327) centre (110.4743, -16.4118) ccw projected
  arc A17 (100.0524, -40.1309) -> (101.1717, -42.9273) centre (101.8338, -41.0401) ccw projected
  line L5 (100.0524, -40.1309) -> (106.107, -28.2683) projected
  arc A18 (108.2854, -27.2173) -> (106.107, -28.2683) centre (107.8884, -29.1775) ccw projected
  arc A19 (108.2854, -27.2173) -> (121.2735, -14.1917) centre (110.4743, -16.4118) ccw projected
  arc A20 (122.3182, -12.0102) -> (121.2735, -14.1917) centre (123.2325, -13.789) ccw projected
  line L6 (122.3182, -12.0102) -> (134.1632, -5.9215) projected
  arc A21 (136.9629, -7.0327) -> (134.1632, -5.9215) centre (135.0776, -7.7003) ccw projected
  line L7 (123.2452, 13.9611) -> (126.1791, 21.9371) projected
  arc A22 (127.9646, 23.2445) -> (126.1791, 21.9371) centre (128.0561, 21.2466) ccw projected
  arc A23 (127.9646, 23.2445) -> (133.0902, 25.8259) centre (127.6431, 30.2622) ccw projected
  arc A24 (136.068, 25.9642) -> (133.0902, 25.8259) centre (134.641, 24.563) ccw projected
  line L8 (136.068, 25.9642) -> (147.8266, 13.9895) projected
  arc A25 (146.3996, 10.5882) -> (147.8266, 13.9895) centre (146.3996, 12.5882) ccw projected
  line L9 (146.3996, 10.5882) -> (138.2732, 10.5882) projected
  arc A26 (138.2732, 10.5882) -> (133.802, 7.8261) centre (138.2732, 5.5882) ccw projected
  arc A27 (130.712, 7.2027) -> (133.802, 7.8261) centre (132.0135, 8.7213) ccw projected
  arc A28 (130.712, 7.2027) -> (124.2371, 11.4772) centre (110.4743, -16.4118) ccw projected
  arc A29 (123.2452, 13.9611) -> (124.2371, 11.4772) centre (125.1222, 13.2707) ccw projected
  arc A30 (74.5837, -8.578) -> (72.0881, -6.2111) centre (70.4743, -10.4118) ccw projected
  arc A31 (70.8888, -3.7727) -> (72.0881, -6.2111) centre (72.8054, -4.3442) ccw projected
  line L10 (70.8888, -3.7727) -> (77.185, 17.3421) projected
  arc A32 (79.524, 18.7255) -> (77.185, 17.3421) centre (79.1016, 16.7706) ccw projected
  arc A33 (79.524, 18.7255) -> (80.8362, 18.6385) centre (80.4743, 23.124) ccw projected
  arc A34 (82.5903, 17.854) -> (80.8362, 18.6385) centre (80.997, 16.645) ccw projected
  line L11 (82.5903, 17.854) -> (89.3833, 8.9018) projected
  arc A35 (89.1607, 6.2363) -> (89.3833, 8.9018) centre (87.79, 7.6928) ccw projected
  arc A36 (89.1607, 6.2363) -> (80.3787, -8.5721) centre (110.4743, -16.4118) ccw projected
  arc A37 (78.1466, -10.0459) -> (80.3787, -8.5721) centre (78.4432, -8.068) ccw projected
  line L12 (78.1466, -10.0459) -> (76.1135, -9.7409) projected
  arc A38 (74.5837, -8.578) -> (76.1135, -9.7409) centre (76.4101, -7.763) ccw projected
  line L13 (103.4349, -26.9045) -> (97.3804, -38.7671) projected
  arc A39 (94.4591, -39.5012) -> (97.3804, -38.7671) centre (95.599, -37.8579) ccw projected
  arc A40 (82.3772, -16.0076) -> (94.4591, -39.5012) centre (110.4743, -16.4118) ccw projected
  arc A41 (84.6737, -14.0585) -> (82.3772, -16.0076) centre (84.377, -16.0364) ccw projected
  line L14 (84.6737, -14.0585) -> (97.8447, -16.0341) projected
  arc A42 (99.5329, -17.7663) -> (97.8447, -16.0341) centre (97.548, -18.012) ccw projected
  arc A43 (99.5329, -17.7663) -> (103.0079, -24.5237) centre (110.4743, -16.4118) ccw projected
  arc A44 (103.4349, -26.9045) -> (103.0079, -24.5237) centre (101.6535, -25.9953) ccw projected
  circle A45 centre (144.4932, -10.0968) radius 1.25 projected
  circle A46 centre (100.1953, 16.6261) radius 1.25 projected
  arc A47 (101.695, -9.7429) -> (100.4118, -11.9067) centre (110.4743, -16.4118) ccw projected
  arc A48 (98.2897, -13.0673) -> (100.4118, -11.9067) centre (98.5864, -11.0895) ccw projected
  line L15 (98.2897, -13.0673) -> (85.1187, -11.0917) projected
  arc A49 (83.4952, -8.5546) -> (85.1187, -11.0917) centre (85.4154, -9.1138) ccw projected
  arc A50 (90.64, 3.4932) -> (83.4952, -8.5546) centre (110.4743, -16.4118) ccw projected
  arc A51 (93.645, 3.2855) -> (90.64, 3.4932) centre (92.0517, 2.0765) ccw projected
  line L16 (93.645, 3.2855) -> (101.6956, -7.3242) projected
  arc A52 (101.695, -9.7429) -> (101.6956, -7.3242) centre (100.1024, -8.5331) ccw projected
  line L17 (116.2133, -5.1551) -> (120.8112, 7.3444) projected
  arc A53 (123.6242, 8.4215) -> (120.8112, 7.3444) centre (122.6883, 6.654) ccw projected
  arc A54 (133.5175, -0.33) -> (123.6242, 8.4215) centre (110.4743, -16.4118) ccw projected
  arc A55 (132.7917, -3.2534) -> (133.5175, -0.33) centre (131.8774, -1.4746) ccw projected
  line L18 (132.7917, -3.2534) -> (120.9467, -9.3421) projected
  arc A56 (118.5647, -8.922) -> (120.9467, -9.3421) centre (120.0323, -7.5633) ccw projected
  arc A57 (118.5647, -8.922) -> (116.9209, -7.468) centre (110.4743, -16.4118) ccw projected
  arc A58 (116.2133, -5.1551) -> (116.9209, -7.468) centre (118.0904, -5.8455) ccw projected
  arc A59 (111.3601, -5.4224) -> (106.4151, -6.1613) centre (110.4743, -16.4118) ccw projected
  arc A60 (104.0855, -5.5107) -> (106.4151, -6.1613) centre (105.6787, -4.3018) ccw projected
  line L19 (104.0855, -5.5107) -> (96.0348, 5.0989) projected
  arc A61 (96.6437, 8.0488) -> (96.0348, 5.0989) centre (97.6281, 6.3079) ccw projected
  arc A62 (116.5511, 11.0233) -> (96.6437, 8.0488) centre (110.4743, -16.4118) ccw projected
  arc A63 (117.9957, 8.3801) -> (116.5511, 11.0233) centre (116.1186, 9.0706) ccw projected
  line L20 (117.9957, 8.3801) -> (113.3978, -4.1194) projected
  arc A64 (111.3601, -5.4224) -> (113.3978, -4.1194) centre (111.5208, -3.4289) ccw projected
  circle A65 centre (94.7451, -47.2298) radius 1.25 projected
  line L21 (123.3635, 22.9728) -> (120.4296, 14.9968) projected
  arc A66 (118.0645, 13.7478) -> (120.4296, 14.9968) centre (118.5526, 15.6873) ccw projected
  arc A67 (118.0645, 13.7478) -> (106.6862, 14.4566) centre (110.4743, -16.4118) ccw projected
  arc A68 (104.4434, 16.5007) -> (106.6862, 14.4566) centre (106.4426, 16.4417) ccw projected
  arc A69 (104.4434, 16.5007) -> (96.7681, 14.1127) centre (100.1953, 16.6261) ccw projected
  arc A70 (96.0809, 11.157) -> (96.7681, 14.1127) centre (95.1553, 12.9299) ccw projected
  arc A71 (96.0809, 11.157) -> (94.4001, 10.212) centre (110.4743, -16.4118) ccw projected
  arc A72 (91.7731, 10.7152) -> (94.4001, 10.212) centre (93.3664, 11.9242) ccw projected
  line L22 (91.7731, 10.7152) -> (84.9801, 19.6674) projected
  arc A73 (84.6967, 21.568) -> (84.9801, 19.6674) centre (86.5734, 20.8764) ccw projected
  arc A74 (84.6967, 21.568) -> (84.9497, 23.594) centre (80.4743, 23.124) ccw projected
  arc A75 (86.5775, 25.77) -> (84.9497, 23.594) centre (86.9388, 23.8029) ccw projected
  line L23 (86.5775, 25.77) -> (118.2794, 31.5925) projected
  arc A76 (120.6357, 29.7665) -> (118.2794, 31.5925) centre (118.6406, 29.6254) ccw projected
  arc A77 (120.6357, 29.7665) -> (122.8508, 25.1256) centre (127.6431, 30.2622) ccw projected
  arc A78 (123.3635, 22.9728) -> (122.8508, 25.1256) centre (121.4865, 23.6632) ccw projected
  arc A79 (117.3199, -46.749) -> (137.4212, -31.9384) centre (110.4743, -16.4118) ccw projected
  line L24 (137.4212, -31.9384) -> (157.6055, 3.092) projected
  arc A80 (157.6055, 3.092) -> (156.8408, 9.0914) centre (153.2732, 5.5882) ccw projected
  line L25 (156.8408, 9.0914) -> (131.9243, 34.466) projected
  arc A81 (131.9243, 34.466) -> (126.5593, 36.1635) centre (127.6431, 30.2622) ccw projected
  line L26 (126.5593, 36.1635) -> (79.6614, 27.5499) projected
  arc A82 (79.6614, 27.5499) -> (76.162, 24.4099) centre (80.4743, 23.124) ccw projected
  line L27 (76.162, 24.4099) -> (66.162, -9.1259) projected
  arc A83 (66.162, -9.1259) -> (66.7172, -12.8885) centre (70.4743, -10.4118) ccw projected
  line L28 (66.7172, -12.8885) -> (90.988, -49.7066) projected
  arc A84 (90.988, -49.7066) -> (95.7356, -51.6195) centre (94.7451, -47.2298) ccw projected
  line L29 (95.7356, -51.6195) -> (117.3199, -46.749) projected
  circle A85 centre (80.4743, 23.124) radius 1.5 projected
  circle A86 centre (138.2732, 5.5882) radius 2 projected
  circle A87 centre (70.4743, -10.4118) radius 1.5 projected
  line L30 (87.7547, -39.351) -> (91.1577, -44.5132)
  line L31 (83.4326, -24.0508) -> (87.7547, -39.351)
  arc A88 (94.4591, -39.5012) -> (97.3804, -38.7671) centre (95.599, -37.8579) ccw projected
  line L32 (97.3804, -38.7671) -> (95.3378, -42.769)
  line L33 (100.0524, -40.1309) -> (98.0099, -44.1329)
  line L34 (116.6595, -43.8226) -> (99.2139, -47.7592)
  line L35 (95.7356, -51.6195) -> (117.3199, -46.749) projected
  line L36 (66.7172, -12.8885) -> (90.988, -49.7066) projected
  arc A89 (101.1717, -42.9273) -> (136.9629, -7.0327) centre (110.4743, -16.4118) ccw projected
  line L37 (100.0524, -40.1309) -> (106.107, -28.2683) projected
  line L38 (103.4349, -26.9045) -> (97.3804, -38.7671) projected
  arc A90 (82.3772, -16.0076) -> (94.4591, -39.5012) centre (110.4743, -16.4118) ccw projected
  line L39 (80.5456, -24.8663) -> (90.0943, -58.6688) construction
  line L40 (78.7483, -25.6886) -> (72.7888, -16.6482) projected
  arc A91 (99.2139, -47.7592) -> (98.0099, -44.1329) centre (94.7451, -47.2298) ccw
  arc A92 (95.3378, -42.769) -> (91.1577, -44.5132) centre (94.7451, -47.2298) ccw
  point P0 (0, 0)
  dimension "d104" = 4.5
  dimension "d105" = 4.5
  constraints: 12 end point, 6 point on circle, 3 collinear, 3 parallel, 3 tangent, 2 centre point, 1 coincident
  measures "d104" radius of A92
  measures "d105" radius of A91
extrude "押し出し15" cut sketch "スケッチ9" against normal blind 2.5 contours A16 L34 A91 L33 A17 | L32 A92 L30 L31 A40 A39
fillet "フィレット2" radius 1 5 edges at (87.7547, -39.351, 1.75) (91.1577, -44.5132, 1.75) (95.3378, -42.769, 1.75) (98.0099, -44.1329, 1.75) (99.2139, -47.7592, 1.75)